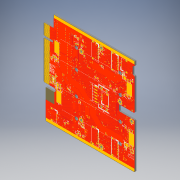
# Autodesk Inventor part: EPS_PCB
Saved by Autodesk Inventor 2018 (Build 220112000, 112)
## iProperties
Created: 2018-01-15
Part Number: EPS_PCB
Material: Epoxy Resin
Document SubType Name: Modeling
Designer: Bradley
Density: 1.14 g/cm^3
Appearance: Smooth - Medium Gray
Mass: 15.4834 g
Surface Area: 175.95 cm^2
Volume: 13.582 cm^3
Author: Bradley
Revision Number: 3.1
Autodesk Inventor part; units mm, degrees
ref_plane "YZ Plane" through (0, 0, 0) normal (1, 0, 0) x (0, 1, 0)
ref_plane "XZ Plane" through (0, 0, 0) normal (0, 1, 0) x (-1, 0, 0)
ref_plane "XY Plane" through (0, 0, 0) normal (0, 0, 1) x (1, 0, 0)
sketch "Sketch1" plane through (0, 0, 0) normal (0, 0, 1) x (1, 0, 0)
  line L0 (0, 36.15) -> (10, 36.15)
  line L1 (10, 36.15) -> (10, 47.9)
  line L2 (10, 47.9) -> (90.4, 47.9)
  line L3 (90.4, 47.9) -> (90.4, -47.9)
  line L4 (90.4, -47.9) -> (2, -47.9)
  line L5 (10, -15.15) -> (0, -15.15)
  line L6 (-5.5, 48) -> (90.5, 48) construction
  line L7 (90.5, 48) -> (90.5, -48) construction
  line L8 (90.5, -48) -> (-5.5, -48) construction
  line L9 (-5.5, -48) -> (-5.5, 48) construction
  line L10 (-5.4, 47.9) -> (-3.4, 47.9) construction
  line L11 (-3.4, 47.9) -> (-3.4, -47.9) construction
  line L12 (-3.4, -47.9) -> (-5.4, -47.9) construction
  line L13 (-5.4, -47.9) -> (-5.4, 47.9) construction
  line L14 (-3.4, 38.5) -> (7.85, 38.5) construction
  line L15 (7.85, 38.5) -> (7.85, -17.5) construction
  line L16 (7.85, -17.5) -> (-3.4, -17.5) construction
  line L17 (-3.4, -17.5) -> (-3.4, 38.5) construction
  line L18 (2, -47.9) -> (2, -18.65)
  line L19 (2, -18.65) -> (10, -18.65)
  arc A0 (10, -18.65) -> (10, -15.15) centre (10, -16.9) ccw
  line L20 (0, 24) -> (90.5, 24) construction
  circle A1 centre (-2.5, 47.1) radius 0.9 construction
  circle A2 centre (-0.7, 47.1) radius 0.9 construction
  circle A3 centre (1.1, 47.1) radius 0.9 construction
  circle A4 centre (2.9, 47.1) radius 0.9 construction
  circle A5 centre (4.7, 47.1) radius 0.9 construction
  circle A6 centre (6.5, 47.1) radius 0.9 construction
  circle A7 centre (8.3, 47.1) radius 0.9 construction
  circle A8 centre (-2.5, 45.3) radius 0.9 construction
  circle A9 centre (-0.7, 45.3) radius 0.9 construction
  circle A10 centre (1.1, 45.3) radius 0.9 construction
  circle A11 centre (2.9, 45.3) radius 0.9 construction
  circle A12 centre (4.7, 45.3) radius 0.9 construction
  circle A13 centre (6.5, 45.3) radius 0.9 construction
  circle A14 centre (8.3, 45.3) radius 0.9 construction
  circle A15 centre (-2.5, 43.5) radius 0.9 construction
  circle A16 centre (-0.7, 43.5) radius 0.9 construction
  circle A17 centre (1.1, 43.5) radius 0.9 construction
  circle A18 centre (2.9, 43.5) radius 0.9 construction
  circle A19 centre (4.7, 43.5) radius 0.9 construction
  circle A20 centre (6.5, 43.5) radius 0.9 construction
  circle A21 centre (8.3, 43.5) radius 0.9 construction
  circle A22 centre (-2.5, 41.7) radius 0.9 construction
  circle A23 centre (-0.7, 41.7) radius 0.9 construction
  circle A24 centre (1.1, 41.7) radius 0.9 construction
  circle A25 centre (2.9, 41.7) radius 0.9 construction
  circle A26 centre (4.7, 41.7) radius 0.9 construction
  circle A27 centre (6.5, 41.7) radius 0.9 construction
  circle A28 centre (8.3, 41.7) radius 0.9 construction
  circle A29 centre (-2.5, 39.9) radius 0.9 construction
  circle A30 centre (-0.7, 39.9) radius 0.9 construction
  circle A31 centre (1.1, 39.9) radius 0.9 construction
  circle A32 centre (2.9, 39.9) radius 0.9 construction
  circle A33 centre (4.7, 39.9) radius 0.9 construction
  circle A34 centre (6.5, 39.9) radius 0.9 construction
  circle A35 centre (8.3, 39.9) radius 0.9 construction
  line L21 (0, 36.15) -> (0, 24.95)
  line L22 (0, 24.95) -> (8.4, 24.95)
  arc A36 (8.4, 23.05) -> (8.4, 24.95) centre (8.4, 24) ccw
  line L23 (8.4, 23.05) -> (0, 23.05)
  line L24 (0, 23.05) -> (0, -15.15)
  point P0 (0, 0)
  point P1 (-5.5, 0)
  point P2 (90.4, 0)
  point P3 (90.5, 0)
  dimension "d0" = 51.3
  dimension "d1" = 95.8
  dimension "d3" = 10
  dimension "d20" = 96
  dimension "d21" = 96
  dimension "d22" = 0.1
  dimension "d23" = 0.1
  dimension "d24" = 2
  dimension "d25" = 0.1
  dimension "d28" = 11.25
  dimension "d29" = 56
  dimension "d31" = 9.5
  dimension "d32" = 30.5
  dimension "d34" = 3.5
  dimension "d35" = 12.15
  dimension "d36" = 39.15
  dimension "d37" = 14.5
  dimension "d38" = 1.15
  dimension "d39" = 1.8
  dimension "d42" = 1.8
  dimension "d45" = 1.8
  dimension "d48" = 2
  dimension "d49" = 3.4
  dimension "d50" = 1.9
  dimension "d51" = 8.4
  dimension "d52" = 24
  constraints: 50 end point, 37 centre point, 11 perpendicular, 7 parallel, 6 point on line, 6 tangent, 5 horizontal, 4 point on circle, 3 midpoint, 3 vertical, 2 collinear, 2 horizontal alignment, 68 other
  measures "d0" distance of L5.end L0.start
  measures "d1" distance of L2.end L3.end
  measures "d3" distance of L0.start L0.end
  measures "d20" distance of L6.start L6.end
  measures "d21" distance of L8.end L6.start
  measures "d22" distance between parallel lines of L2 L6
  measures "d23" distance between parallel lines of L7 L3
  measures "d24" distance between parallel lines of L13 L11
  measures "d25" distance between parallel lines of L13 L9
  measures "d28" distance of L15.end L16.end
  measures "d29" distance of L14.end L15.end
  measures "d31" distance between parallel lines of L14 L6
  measures "d32" distance between parallel lines of L8 L16
  measures "d34" distance between parallel lines of L5 L19
  measures "d35" distance between parallel lines of L20 L0
  measures "d36" distance between parallel lines of L5 L20
  measures "d37" distance between parallel lines of L20 L14
  measures "d38" distance between parallel lines of L19 L16
  measures "d39" diameter of A1
  measures "d42" distance of A1.centre A2.centre
  measures "d45" distance of A1.centre A8.centre
  measures "d48" distance between parallel lines of L18 L24
  measures "d49" distance between parallel lines of L24 L11
  measures "d50" distance between parallel lines of L23 L22
  measures "d51" distance of L21.end L22.end
  measures "d52" distance from line of point (0, 0) L20
extrude "Extrusion1" add sketch "Sketch1" along normal mid plane 1.6
chamfer "Chamfer1" distance 0.5 angle 45 4 edges at (0, 36.15, 0) (0, 24.95, 0) (0, 23.05, 0) (0, -15.15, 0)
fillet "Fillet1" radius 0.5 6 edges at (10, 36.15, 0) (10, 47.9, 0) (90.4, 47.9, 0) (90.4, -47.9, 0) (2, -47.9, 0) (2, -18.65, 0)
sketch "Sketch6" plane through (0, 0, 0.8) normal (0, 0, 1) x (1, 0, 0)
  arc A0 (2.5, -18.65) -> (2, -19.15) centre (2.5, -19.15) ccw projected
  line L0 (2, -19.15) -> (2, -47.4) projected
  arc A1 (2, -47.4) -> (2.5, -47.9) centre (2.5, -47.4) ccw projected
  line L1 (2.5, -47.9) -> (89.9, -47.9) projected
  arc A2 (89.9, -47.9) -> (90.4, -47.4) centre (89.9, -47.4) ccw projected
  line L2 (90.4, -47.4) -> (90.4, 47.4) projected
  arc A3 (90.4, 47.4) -> (89.9, 47.9) centre (89.9, 47.4) ccw projected
  line L3 (89.9, 47.9) -> (10.5, 47.9) projected
  arc A4 (10.5, 47.9) -> (10, 47.4) centre (10.5, 47.4) ccw projected
  line L4 (10, 47.4) -> (10, 36.65) projected
  arc A5 (9.5, 36.15) -> (10, 36.65) centre (9.5, 36.65) ccw projected
  line L5 (9.5, 36.15) -> (0.5, 36.15) projected
  line L6 (0, 35.65) -> (0.5, 36.15) projected
  line L7 (0, 35.65) -> (0, 25.45) projected
  line L8 (0.5, 24.95) -> (0, 25.45) projected
  line L9 (0.5, 24.95) -> (8.4, 24.95) projected
  arc A6 (8.4, 23.05) -> (8.4, 24.95) centre (8.4, 24) ccw projected
  line L10 (8.4, 23.05) -> (0.5, 23.05) projected
  line L11 (0, 22.55) -> (0.5, 23.05) projected
  line L12 (0, 22.55) -> (0, -14.65) projected
  line L13 (0.5, -15.15) -> (0, -14.65) projected
  line L14 (0.5, -15.15) -> (10, -15.15) projected
  arc A7 (10, -18.65) -> (10, -15.15) centre (10, -16.9) ccw projected
  line L15 (10, -18.65) -> (2.5, -18.65) projected
  line L16 (90.4, 47.4) -> (90.4, -47.4) projected
  arc A8 (89.4, 3) -> (90.4, 4) centre (89.4, 4) ccw
  line L17 (89.4, 3) -> (75.9, 3)
  arc A9 (75.9, 3) -> (74.9, 2) centre (75.9, 2) ccw
  line L18 (74.9, 2) -> (74.9, -2)
  arc A10 (74.9, -2) -> (75.9, -3) centre (75.9, -2) ccw
  line L19 (75.9, -3) -> (89.4, -3)
  arc A11 (90.4, -4) -> (89.4, -3) centre (89.4, -4) ccw
  arc A12 (90.4, 34) -> (89.4, 35) centre (89.4, 34) ccw
  arc A13 (88.4, 36) -> (89.4, 35) centre (89.4, 36) ccw
  line L20 (88.4, 36) -> (88.4, 42)
  arc A14 (89.4, 43) -> (88.4, 42) centre (89.4, 42) ccw
  arc A15 (89.4, 43) -> (90.4, 44) centre (89.4, 44) ccw
  point P0 (0, 0)
  point P1 (74.9, 0)
  dimension "d69" = 6
  dimension "d70" = 1
  dimension "d71" = 15.5
  dimension "d81" = 2
  dimension "d82" = 35
  dimension "d83" = 8
  constraints: 16 point on circle, 14 tangent, 8 centre point, 8 end point, 6 equal radius, 4 point on line, 2 perpendicular, 1 horizontal, 1 horizontal alignment, 1 midpoint, 1 vertical, 1 vertical alignment
  measures "d69" distance between parallel lines of L19 L17
  measures "d70" radius of A8
  measures "d71" distance between parallel lines of L2 L18
  measures "d81" distance between parallel lines of L16 L20
  measures "d82" vertical distance of point (0, 0) A12.end
  measures "d83" distance of A12.end A14.start
extrude "Extrusion5" cut sketch "Sketch6" against normal through all contours A11 L19 A10 L18 A9 L17 A8 L2 | A12 A13 L20 A14 A15 L2
sketch "Sketch7" plane through (0, 0, 0.8) normal (0, 0, 1) x (1, 0, 0)
  point P0 (0, 0)
  point P1 (76, -30.5)
  point P2 (32.5, 30.5)
  point P3 (76, 30.5)
  point P4 (76, 11.5)
  point P5 (32.5, 11.5)
  point P6 (76, -11.5)
  point P7 (32.5, -11.5)
  point P8 (32.5, -30.5)
  constraints: 8 other
hole "Hole2" at (76, -30.5, 0.8) at (32.5, 30.5, 0.8) at (76, 30.5, 0.8) at (76, 11.5, 0.8) at (32.5, 11.5, 0.8) at (76, -11.5, 0.8) at (32.5, -11.5, 0.8) at (32.5, -30.5, 0.8) direction (0, 0, -1) diameter 3 end through all
sketch "Sketch8" plane through (0, 0, 0.8) normal (0, 0, 1) x (1, 0, 0)
  point P0 (0, 0)
  point P1 (37.4, -29.6)
  point P2 (57.3, -42.5)
  point P3 (87.4, -5.5)
  point P4 (75.9, 5.5)
  point P5 (37.4, 29.6)
  point P6 (57.3, 42.5)
  constraints: 6 other
hole "Hole3" at (37.4, -29.6, 0.8) at (57.3, -42.5, 0.8) at (87.4, -5.5, 0.8) at (75.9, 5.5, 0.8) at (37.4, 29.6, 0.8) at (57.3, 42.5, 0.8) direction (0, 0, -1) diameter 2.2 end through all
sketch "Sketch9" plane through (0, 0, 0.8) normal (0, 0, 1) x (1, 0, 0)
  point P0 (0, 0)
  point P1 (62.54, 8)
  point P2 (57.46, 8)
  point P3 (62.54, -8)
  point P4 (57.46, -8)
  constraints: 4 other
hole "Hole4" at (62.54, 8, 0.8) at (57.46, 8, 0.8) at (62.54, -8, 0.8) at (57.46, -8, 0.8) direction (0, 0, -1) diameter 1.2 end through all
sketch "Sketch10" plane through (0, 0, 0.8) normal (0, 0, 1) x (1, 0, 0)
  point P0 (0, 0)
  point P1 (7.9, 9.6)
  point P2 (12.3, -3.9)
  constraints: 2 other
hole "Hole5" at (7.9, 9.6, 0.8) at (12.3, -3.9, 0.8) direction (0, 0, -1) diameter 1 end through all
sketch "Sketch11" plane through (0, 0, 0.8) normal (0, 0, 1) x (1, 0, 0)
  point P0 (0, 0)
  point P1 (87.975, 4.15)
  point P2 (80.725, 4.15)
  point P3 (34.1, 39.2)
  point P4 (36.1, -33.4)
  constraints: 4 other
hole "Hole6" at (87.975, 4.15, 0.8) at (80.725, 4.15, 0.8) at (34.1, 39.2, 0.8) at (36.1, -33.4, 0.8) direction (0, 0, -1) diameter 0.7 end through all
sketch "Sketch12" plane through (0, 0, 0.8) normal (0, 0, 1) x (1, 0, 0)
  point P0 (0, 0)
  point P1 (58.431, -41.369)
  point P2 (57.3, -40.9)
  point P3 (56.169, -41.369)
  point P4 (55.7, -42.5)
  point P5 (56.169, -43.631)
  point P6 (57.3, -44.1)
  point P7 (58.431, -43.631)
  point P8 (77.5, 5.5)
  point P9 (77.031, 6.631)
  point P10 (75.9, 7.1)
  point P11 (74.769, 6.631)
  point P12 (74.3, 5.5)
  point P13 (74.769, 4.369)
  point P14 (75.9, 3.9)
  point P15 (77.031, 4.369)
  point P16 (87.4, -3.9)
  point P17 (86.269, -4.369)
  point P18 (85.8, -5.5)
  point P19 (86.269, -6.631)
  point P20 (87.4, -7.1)
  point P21 (88.531, -6.631)
  point P22 (89, -5.5)
  point P23 (39, 29.6)
  point P24 (38.531, 30.731)
  point P25 (37.4, 31.2)
  point P26 (36.269, 30.731)
  point P27 (35.8, 29.6)
  point P28 (36.269, 28.469)
  point P29 (37.4, 28)
  point P30 (39, -29.6)
  point P31 (88.531, -4.369)
  point P32 (58.9, 42.5)
  point P33 (58.431, 43.631)
  point P34 (38.531, -28.469)
  point P35 (56.169, 43.631)
  point P36 (55.7, 42.5)
  point P37 (56.169, 41.369)
  point P38 (57.3, 40.9)
  point P39 (38.531, 28.469)
  point P40 (37.4, -28)
  point P41 (57.3, 44.1)
  point P42 (36.269, -28.469)
  point P43 (35.8, -29.6)
  point P44 (36.269, -30.731)
  point P45 (37.4, -31.2)
  point P46 (38.531, -30.731)
  point P47 (58.9, -42.5)
  point P48 (58.431, 41.369)
  constraints: 48 other
hole "Hole7" at (58.431, -41.369, 0.8) at (57.3, -40.9, 0.8) at (56.169, -41.369, 0.8) at (55.7, -42.5, 0.8) at (56.169, -43.631, 0.8) at (57.3, -44.1, 0.8) at (58.431, -43.631, 0.8) at (77.5, 5.5, 0.8) at (77.031, 6.631, 0.8) at (75.9, 7.1, 0.8) at (74.769, 6.631, 0.8) at (74.3, 5.5, 0.8) at (74.769, 4.369, 0.8) at (75.9, 3.9, 0.8) at (77.031, 4.369, 0.8) at (87.4, -3.9, 0.8) at (86.269, -4.369, 0.8) at (85.8, -5.5, 0.8) at (86.269, -6.631, 0.8) at (87.4, -7.1, 0.8) at (88.531, -6.631, 0.8) at (89, -5.5, 0.8) at (39, 29.6, 0.8) at (38.531, 30.731, 0.8) at (37.4, 31.2, 0.8) at (36.269, 30.731, 0.8) at (35.8, 29.6, 0.8) at (36.269, 28.469, 0.8) at (37.4, 28, 0.8) at (39, -29.6, 0.8) at (88.531, -4.369, 0.8) at (58.9, 42.5, 0.8) at (58.431, 43.631, 0.8) at (38.531, -28.469, 0.8) at (56.169, 43.631, 0.8) at (55.7, 42.5, 0.8) at (56.169, 41.369, 0.8) at (57.3, 40.9, 0.8) at (38.531, 28.469, 0.8) at (37.4, -28, 0.8) at (57.3, 44.1, 0.8) at (36.269, -28.469, 0.8) at (35.8, -29.6, 0.8) at (36.269, -30.731, 0.8) at (37.4, -31.2, 0.8) at (38.531, -30.731, 0.8) at (58.9, -42.5, 0.8) at (58.431, 41.369, 0.8) direction (0, 0, -1) diameter 0.35 end through all
sketch "Sketch13" plane through (0, 0, 0.8) normal (0, 0, 1) x (1, 0, 0)
  point P0 (0, 0)
  point P1 (13.9, 37.7)
  point P2 (13.9, 41.7)
  point P3 (13.9, 33.7)
  point P4 (13.9, 29.7)
  point P5 (16, 25.7)
  point P6 (16, 21.7)
  point P7 (16, 17.7)
  point P8 (15.9, 13.7)
  point P9 (16, 9.7)
  point P10 (15.9, 5.7)
  point P11 (23.7, 3.7)
  point P12 (23.7, 7.7)
  point P13 (23.915, 11.745)
  point P14 (23.7, 15.7)
  point P15 (23.765, 19.74)
  point P16 (23.7, 23.7)
  point P17 (23.7, 27.7)
  point P18 (21.69, 31.695)
  point P19 (21.7, 35.7)
  point P20 (21.7, 39.7)
  point P21 (10.29, 10.02)
  point P22 (12.8, -10.8)
  point P23 (37.7, 36.5)
  point P24 (52.5, 35.9)
  point P25 (51.3, 31.8)
  point P26 (51.4, 43.8)
  point P27 (51.4, 43)
  point P28 (51.4, 42.2)
  point P29 (52.2, 42.2)
  point P30 (35.2, 40.4)
  point P31 (35.2, 39.6)
  point P32 (35.2, 38.8)
  point P33 (36.9, 40.4)
  point P34 (36.9, 39.6)
  point P35 (36.9, 38.8)
  point P36 (39.7, 31.6)
  point P37 (39.7, 30.8)
  point P38 (41.8, 35.2)
  point P39 (42.1, 35.8)
  point P40 (41.8, 36.4)
  point P41 (40.8, 36.5)
  point P42 (39.8, 36.4)
  point P43 (39.5, 35.8)
  point P44 (39.8, 35.2)
  point P45 (43.2, 19.5)
  point P46 (43.2, 20.7)
  point P47 (44.8, 19.5)
  point P48 (44, 19.5)
  point P49 (40.5, 31.6)
  point P50 (40.5, 30)
  point P51 (57.2, 36)
  point P52 (57.2, 38.9)
  point P53 (64.8, 40.7)
  point P54 (61.95, 43.2)
  point P55 (59.3, 30.1)
  point P56 (68.2, 36.7)
  point P57 (71, 36.7)
  point P58 (73.5, 33)
  point P59 (63.6, 30.8)
  point P60 (64.2, 32.9)
  point P61 (66.6, 31.9)
  point P62 (69.7, 29.7)
  point P63 (10.6, 42)
  point P64 (22, 18.695)
  point P65 (22, 9.7)
  point P66 (29.47, 15.2)
  point P67 (40, 22.6)
  point P68 (35.3, 27.2)
  point P69 (39.4, 27.1)
  point P70 (46.6, -43.1)
  point P71 (46.6, -44.4)
  point P72 (47.4, -44.4)
  point P73 (47.4, -43.7)
  point P74 (47.4, -43)
  point P75 (46.6, -43.7)
  point P76 (42.2, -37.8)
  point P77 (41.6, -37.8)
  point P78 (41, -37.8)
  point P79 (40.9, -38.8)
  point P80 (41, -39.8)
  point P81 (41.6, -40.1)
  point P82 (42.2, -39.8)
  point P83 (41.6, -35.4)
  point P84 (42.4, -35.4)
  point P85 (43.2, -35.4)
  point P86 (42.4, -37.1)
  point P87 (41.7, -37.1)
  point P88 (50.2, -28.8)
  point P89 (51, -28.8)
  point P90 (51.8, -28.8)
  point P91 (52.6, -28.8)
  point P92 (52.6, -28)
  point P93 (52.6, -27.2)
  point P94 (53.1, -31.5)
  point P95 (57.6, -40)
  point P96 (64.8, -42.9)
  point P97 (64.7, -39.8)
  point P98 (73.8, -42.9)
  point P99 (73.5, -40.62)
  point P100 (68.2, -38.9)
  point P101 (64.7, -34.7)
  point P102 (70.1, -34.7)
  point P103 (60, -34.6)
  point P104 (12, -41.3)
  point P105 (6.7, -40.65)
  point P106 (79.8, -31.7)
  point P107 (84.6, -33)
  point P108 (59.1, -32.9)
  point P109 (82.75, -5.8)
  point P110 (89.4, -37.7)
  point P111 (54, 33)
  point P112 (77.9, 41.2)
  point P113 (77.7, 35)
  point P114 (43.2, 20.1)
  point P115 (45.6, 20.1)
  point P116 (83.2, 10.9)
  point P117 (78.415, 10.635)
  point P118 (82, 13.8)
  point P119 (58, 1.5)
  point P120 (35.7, -24.95)
  point P121 (38.2, -15.4)
  point P122 (45.6, 19.5)
  point P123 (52.2, 43)
  point P124 (41, -36.2)
  point P125 (41, -37)
  point P126 (6.1, 11.1)
  point P127 (6.1, 10.3)
  point P128 (6.1, 9.5)
  point P129 (6.1, 8.7)
  point P130 (6.1, 7.9)
  point P131 (6.1, 7.1)
  point P132 (6.1, 6.3)
  point P133 (6.1, 5.5)
  point P134 (78.29, -34.2)
  point P135 (87.1, 36.4)
  point P136 (77.34, 13.12)
  point P137 (71.66, -8.115)
  point P138 (85.155, -30.25)
  point P139 (72.8, -18.24)
  point P140 (72.76, -19.96)
  point P141 (78.29, -35)
  point P142 (87.095, 35.64)
  point P143 (77.335, 13.88)
  point P144 (71.4, -7.4)
  point P145 (85.155, -31.015)
  point P146 (72.04, -18.24)
  point P147 (72, -19.96)
  point P148 (81.78, -23.295)
  point P149 (66, -2.185)
  point P150 (69.9, -2.2)
  point P151 (56.6, 33.9)
  point P152 (70, 28.3)
  point P153 (68.4, 33.9)
  point P154 (62, 39.1)
  point P155 (60.9, 32.5)
  point P156 (71.39, -36.73)
  point P157 (62.5, -35.8)
  point P158 (62.8, -39.2)
  point P159 (67.1, -32.9)
  point P160 (81.5, 15.2)
  point P161 (81.8, 16.99)
  point P162 (81.2, 16.99)
  point P163 (80.6, 16.99)
  point P164 (81.8, 17.59)
  point P165 (81.2, 17.59)
  point P166 (82.1, 15.2)
  point P167 (82.1, 14.6)
  point P168 (81.5, 14.6)
  point P169 (68.2, 2)
  point P170 (56.4, 36.81)
  point P171 (62, 33.1)
  point P172 (69, 28.1)
  point P173 (74.5, 37.3)
  point P174 (71.18, 27.71)
  point P175 (72.5, 34.9)
  point P176 (72, 27.6)
  point P177 (58, -36.75)
  point P178 (38.7, -35.5)
  point P179 (59.1, -39.8)
  point P180 (38.7, -41.5)
  point P181 (75, -37.9)
  point P182 (37.8, -35.6)
  point P183 (75.5, -41.6)
  point P184 (70.2, -37.9)
  point P185 (37.86, -38.715)
  point P186 (68.5, 37.65)
  point P187 (66.3, -43.2)
  point P188 (66.3, -36.73)
  point P189 (84.3, -15)
  point P190 (82.7, -15.8)
  point P191 (83.5, -15.8)
  point P192 (83.5, -15)
  point P193 (84.3, -14.2)
  point P194 (83.5, -14.2)
  point P195 (82.7, -15)
  point P196 (82.7, -14.2)
  point P197 (65.6, 33.5)
  point P198 (84.5, 13.8)
  point P199 (70.7, -4.8)
  constraints: 687 other
hole "Hole8" at (13.9, 37.7, 0.8) at (13.9, 41.7, 0.8) at (13.9, 33.7, 0.8) at (13.9, 29.7, 0.8) at (16, 25.7, 0.8) at (16, 21.7, 0.8) at (16, 17.7, 0.8) at (15.9, 13.7, 0.8) at (16, 9.7, 0.8) at (15.9, 5.7, 0.8) at (23.7, 3.7, 0.8) at (23.7, 7.7, 0.8) at (23.915, 11.745, 0.8) at (23.7, 15.7, 0.8) at (23.765, 19.74, 0.8) at (23.7, 23.7, 0.8) at (23.7, 27.7, 0.8) at (21.69, 31.695, 0.8) at (21.7, 35.7, 0.8) at (21.7, 39.7, 0.8) at (10.29, 10.02, 0.8) at (12.8, -10.8, 0.8) at (37.7, 36.5, 0.8) at (52.5, 35.9, 0.8) at (51.3, 31.8, 0.8) at (51.4, 43.8, 0.8) at (51.4, 43, 0.8) at (51.4, 42.2, 0.8) at (52.2, 42.2, 0.8) at (35.2, 40.4, 0.8) at (35.2, 39.6, 0.8) at (35.2, 38.8, 0.8) at (36.9, 40.4, 0.8) at (36.9, 39.6, 0.8) at (36.9, 38.8, 0.8) at (39.7, 31.6, 0.8) at (39.7, 30.8, 0.8) at (41.8, 35.2, 0.8) at (42.1, 35.8, 0.8) at (41.8, 36.4, 0.8) at (40.8, 36.5, 0.8) at (39.8, 36.4, 0.8) at (39.5, 35.8, 0.8) at (39.8, 35.2, 0.8) at (43.2, 19.5, 0.8) at (43.2, 20.7, 0.8) at (44.8, 19.5, 0.8) at (44, 19.5, 0.8) at (40.5, 31.6, 0.8) at (40.5, 30, 0.8) direction (0, 0, -1) diameter 0.3 end through all and at (57.2, 36, 0.8) (57.2, 38.9, 0.8) (64.8, 40.7, 0.8) (61.95, 43.2, 0.8) (59.3, 30.1, 0.8) (68.2, 36.7, 0.8) (71, 36.7, 0.8) (73.5, 33, 0.8) (63.6, 30.8, 0.8) (64.2, 32.9, 0.8) (66.6, 31.9, 0.8) (69.7, 29.7, 0.8) (10.6, 42, 0.8) (22, 18.695, 0.8) (22, 9.7, 0.8) (29.47, 15.2, 0.8) (40, 22.6, 0.8) (35.3, 27.2, 0.8) (39.4, 27.1, 0.8) (46.6, -43.1, 0.8) (46.6, -44.4, 0.8) (47.4, -44.4, 0.8) (47.4, -43.7, 0.8) (47.4, -43, 0.8) (46.6, -43.7, 0.8) (42.2, -37.8, 0.8) (41.6, -37.8, 0.8) (41, -37.8, 0.8) (40.9, -38.8, 0.8) (41, -39.8, 0.8) (41.6, -40.1, 0.8) (42.2, -39.8, 0.8) (41.6, -35.4, 0.8) (42.4, -35.4, 0.8) (43.2, -35.4, 0.8) (42.4, -37.1, 0.8) (41.7, -37.1, 0.8) (50.2, -28.8, 0.8) (51, -28.8, 0.8) (51.8, -28.8, 0.8) (52.6, -28.8, 0.8) (52.6, -28, 0.8) (52.6, -27.2, 0.8) (53.1, -31.5, 0.8) (57.6, -40, 0.8) (64.8, -42.9, 0.8) (64.7, -39.8, 0.8) (73.8, -42.9, 0.8) (73.5, -40.62, 0.8) (68.2, -38.9, 0.8) (64.7, -34.7, 0.8) (70.1, -34.7, 0.8) (60, -34.6, 0.8) (12, -41.3, 0.8) (6.7, -40.65, 0.8) (79.8, -31.7, 0.8) (84.6, -33, 0.8) (59.1, -32.9, 0.8) (82.75, -5.8, 0.8) (89.4, -37.7, 0.8) (54, 33, 0.8) (77.9, 41.2, 0.8) (77.7, 35, 0.8) (43.2, 20.1, 0.8) (45.6, 20.1, 0.8) (83.2, 10.9, 0.8) (78.415, 10.635, 0.8) (82, 13.8, 0.8) (58, 1.5, 0.8) (35.7, -24.95, 0.8) (38.2, -15.4, 0.8) (45.6, 19.5, 0.8) (52.2, 43, 0.8) (41, -36.2, 0.8) (41, -37, 0.8) (6.1, 11.1, 0.8) (6.1, 10.3, 0.8) (6.1, 9.5, 0.8) (6.1, 8.7, 0.8) (6.1, 7.9, 0.8) (6.1, 7.1, 0.8) (6.1, 6.3, 0.8) (6.1, 5.5, 0.8) (78.29, -34.2, 0.8) (87.1, 36.4, 0.8) (77.34, 13.12, 0.8) (71.66, -8.115, 0.8) (85.155, -30.25, 0.8) (72.8, -18.24, 0.8) (72.76, -19.96, 0.8) (78.29, -35, 0.8) (87.095, 35.64, 0.8) (77.335, 13.88, 0.8) (71.4, -7.4, 0.8) (85.155, -31.015, 0.8) (72.04, -18.24, 0.8) (72, -19.96, 0.8) (81.78, -23.295, 0.8) (66, -2.185, 0.8) (69.9, -2.2, 0.8) (56.6, 33.9, 0.8) (70, 28.3, 0.8) (68.4, 33.9, 0.8) (62, 39.1, 0.8) (60.9, 32.5, 0.8) (71.39, -36.73, 0.8) (62.5, -35.8, 0.8) (62.8, -39.2, 0.8) (67.1, -32.9, 0.8) (81.5, 15.2, 0.8) (81.8, 16.99, 0.8) (81.2, 16.99, 0.8) (80.6, 16.99, 0.8) (81.8, 17.59, 0.8) (81.2, 17.59, 0.8) (82.1, 15.2, 0.8) (82.1, 14.6, 0.8) (81.5, 14.6, 0.8) (68.2, 2, 0.8) (56.4, 36.81, 0.8) (62, 33.1, 0.8) (69, 28.1, 0.8) (74.5, 37.3, 0.8) (71.18, 27.71, 0.8) (72.5, 34.9, 0.8) (72, 27.6, 0.8) (58, -36.75, 0.8) (38.7, -35.5, 0.8) (59.1, -39.8, 0.8) (38.7, -41.5, 0.8) (75, -37.9, 0.8) (37.8, -35.6, 0.8) (75.5, -41.6, 0.8) (70.2, -37.9, 0.8) (37.86, -38.715, 0.8) (68.5, 37.65, 0.8) (66.3, -43.2, 0.8) (66.3, -36.73, 0.8) (84.3, -15, 0.8) (82.7, -15.8, 0.8) (83.5, -15.8, 0.8) (83.5, -15, 0.8) (84.3, -14.2, 0.8) (83.5, -14.2, 0.8) (82.7, -15, 0.8) (82.7, -14.2, 0.8) (65.6, 33.5, 0.8) (84.5, 13.8, 0.8) (70.7, -4.8, 0.8) (83.355, -3.96, 0.8) (77, 37.5, 0.8) (5.3, -38.3, 0.8) (18.7, -43.7, 0.8) (81.7, -33.4, 0.8) (87.2, -34.6, 0.8) (67.3, 19.215, 0.8) (65.34, 16.795, 0.8) (58.84, -22.08, 0.8) (71.54, -11.46, 0.8) (53.71, -6.57, 0.8) (68, 18.915, 0.8) (65.88, 16.255, 0.8) (58.08, -22.08, 0.8) (71.76, -12.19, 0.8) (54.345, -6.99, 0.8) (69.5, 19.215, 0.8) (66.96, 15.175, 0.8) (72.94, -11.7, 0.8) (59.17, -23.16, 0.8) (53.89, -5.83, 0.8) (68.8, 18.915, 0.8) (66.42, 15.715, 0.8) (59.93, -23.17, 0.8) (72.62, -11.01, 0.8) (54.57, -5.49, 0.8) (8.09, -8.99, 0.8) (6.2, -11.2, 0.8) (22.4, -12.1, 0.8) (22.4, -15, 0.8) (29.8, 34.1, 0.8) (34.9, 32.9, 0.8) (36.025, 15.595, 0.8) (28.5, -39.9, 0.8) (29.2, -42.7, 0.8) (13.9, -44, 0.8) (80.1, -35.8, 0.8) (77.395, -37.24, 0.8) (80.3, -11.5, 0.8) (78.1, -11.1, 0.8) (61.465, -22.4, 0.8) (47.7, 6.3, 0.8) (36.1, 2.8, 0.8) (22.6, -0.4, 0.8) (77.6, 23.5, 0.8) (63.7, 13.27, 0.8) (51.395, 20.445, 0.8) (44.8, 13.3, 0.8) (46.1, -10.8, 0.8) (38.1, -9.9, 0.8) (50.3, 2, 0.8) (61.82, -4.17, 0.8) (44.5, -14.6, 0.8) (24.9, -17.7, 0.8) (28.4, -18.5, 0.8) (64.69, 33.91, 0.8) (55.96, 26.7, 0.8) (39.3, -25.44, 0.8) (20.7, -36.8, 0.8) (16, 14.5, 0.8) (16, 10.5, 0.8) (16, 6.5, 0.8) (23.8, 4.5, 0.8) (23.8, 8.5, 0.8) (23.8, 12.5, 0.8) (23.8, 16.5, 0.8) (27.1, 15.2, 0.8) (52.3, -41.5, 0.8) (53, -41.5, 0.8) (53, -42.3, 0.8) (55, -40.3, 0.8) (55.8, -40.3, 0.8) (55, -41.1, 0.8) (62.8, -29, 0.8) (62.8, -29.8, 0.8) (61.9, -29.8, 0.8) (61.9, -29, 0.8) (61.9, -28.2, 0.8) (61.1, -29, 0.8) (61.1, -28.2, 0.8) (81.5, -26.1, 0.8) (81.2, 25.9, 0.8) (61, 12.46, 0.8) (51.3, -13.2, 0.8) (4.3, -36.6, 0.8) (61.1, -29.8, 0.8) (52.3, -42.3, 0.8) (53.8, -42.3, 0.8) (11.795, 7.67, 0.8) (12.3, 7.1, 0.8) (16, 15.98, 0.8) (15.995, 11.98, 0.8) (16, 7.98, 0.8) (23.8, 6, 0.8) (23.8, 10, 0.8) (23.8, 14, 0.8) (23.9, 18, 0.8) (45.9, 25, 0.8) (46.7, 25, 0.8) (47.5, 25, 0.8) (48.3, 25, 0.8) (48.3, 25.8, 0.8) (48.3, 26.6, 0.8) (82, -4.3, 0.8) (73.9, 28.4, 0.8) (64.22, 18.4, 0.8) (6.8, -39.2, 0.8) (13.7, 4.4, 0.8) (56.315, 27.375, 0.8) (40.7, -42.7, 0.8) (34.9, -39.7, 0.8) (83.9, -22.5, 0.8) (83.9, -17.2, 0.8) (82.4, -25.6, 0.8) (20.9, -41.7, 0.8) (24, -42.8, 0.8) (36.2, -35.4, 0.8) (81.9, 23.3, 0.8) (44.1, 22.1, 0.8) (54.4, 15.9, 0.8) (52.5, 14.6, 0.8) (26.7, -4.3, 0.8) (46.3, 19.8, 0.8) (71.18, 17.96, 0.8) (75.1, 17.3, 0.8) (71.66, 12.95, 0.8) (61, 18.735, 0.8) (65.465, 13.585, 0.8) (71.28, -18.24, 0.8) (36, 4.7, 0.8) (50.4, 11.1, 0.8) (89.8, 14.2, 0.8) (83, -24.1, 0.8) (82.2, -24.1, 0.8) (85.2, 28.9, 0.8) (84.4, 28.9, 0.8) (85.6, -29.1, 0.8) (88.6, 28.4, 0.8) (88.4, 13, 0.8) (81, 31.3, 0.8) (81.5, -31.5, 0.8) (87.2, -28.8, 0.8) (86.4, -28.8, 0.8) (88.3, -31.1, 0.8) (88.2, -12.7, 0.8) (87.4, -12.7, 0.8) (15.4, -11, 0.8) (15.4, -12.6, 0.8) (17, -12.91, 0.8) (15.45, -35.315, 0.8) (89.4, -31.4, 0.8) (87.3, 12.1, 0.8) (85.6, 12.1, 0.8) (69.8, 2.8, 0.8) (79.6, 11.8, 0.8) (5.9, -5.5, 0.8) (39.69, -0.55, 0.8) (78.82, 13.46, 0.8) (41.7, 39.2, 0.8) (14, 44, 0.8) (14.005, 39.975, 0.8) (14, 35.98, 0.8) (14.005, 31.98, 0.8) (16.005, 27.98, 0.8) (16, 23.98, 0.8) (16, 19.98, 0.8) (23.9, 22, 0.8) (23.8, 26, 0.8) (21.8, 34, 0.8) (21.8, 38, 0.8) (21.8, 42, 0.8) (23.58, 30.6, 0.8) (37.5, 42.4, 0.8) (36.7, 42.4, 0.8) (36.7, 43.2, 0.8) (37.5, 43.2, 0.8) (37.5, 41.6, 0.8) (36.7, 41.6, 0.8) (58.69, 28.175, 0.8) (48.935, 19.86, 0.8) (44.92, 10.98, 0.8) (57.11, -21.28, 0.8) (38.9, 2.5, 0.8) (38.9, 4.2, 0.8) (49.9, -10.235, 0.8) (83, -37, 0.8) (89.2, -34.7, 0.8) (14, 42.5, 0.8) (14, 38.5, 0.8) (14, 34.5, 0.8) (14, 30.5, 0.8) (16, 26.5, 0.8) (16, 22.5, 0.8) (16, 18.5, 0.8) (23.815, 20.5, 0.8) (23.8, 24.5, 0.8) (23.8, 28.5, 0.8) (21.765, 32.54, 0.8) (21.8, 36.5, 0.8) (21.8, 40.5, 0.8) (13, 44.4, 0.8) (42.9, -22.6, 0.8) (42.3, -22.9, 0.8) (43.7, -22.6, 0.8) (43.7, -23.4, 0.8) (43.7, -24.2, 0.8) (88, -34.7, 0.8) (18.5, 1.1, 0.8) (19.3, 1.1, 0.8) (20.1, 1.1, 0.8) (20.1, 0.3, 0.8) (19.3, 0.3, 0.8) (18.5, 0.3, 0.8) (18.5, -0.5, 0.8) (19.3, -0.5, 0.8) (42.295, -15.04, 0.8) (44.5, -22.6, 0.8) (44.5, -23.4, 0.8) (44.5, -24.2, 0.8) (45.3, -24.2, 0.8) (45.3, -23.4, 0.8) (45.3, -22.6, 0.8) (42.9, -27.9, 0.8) (39.9, -33.9, 0.8) (30, 39.4, 0.8) (74.765, 16.16, 0.8) (72.8, 16.2, 0.8) (39.2, -44, 0.8) (32.1, -44.4, 0.8) (28.855, -9.895, 0.8) (30.815, -16.8, 0.8) (39.98, -26.8, 0.8) (17.6, -37.7, 0.8) (5.9, 35.5, 0.8) (9.55, -9.34, 0.8) (10.1, -6.5, 0.8) (5.9, 34.5, 0.8) (12.1, 40.835, 0.8) (5.9, 33.5, 0.8) (11.7, 39.45, 0.8) (5.9, 32.5, 0.8) (5.9, 31.5, 0.8) (5.9, 30.5, 0.8) (5.9, 29.5, 0.8) (5.9, 28.5, 0.8) (5.9, 27.5, 0.8) (5.9, 26.5, 0.8) (5.9, 25.6, 0.8) (9.3, 25.5, 0.8) (5.9, 22.4, 0.8) (9.1, 22.5, 0.8) (5.9, 21.5, 0.8) (28.03, 40.835, 0.8) (33.84, 20.76, 0.8) (27.615, 38.87, 0.8) (33.67, 20.015, 0.8) (25.8, 39.1, 0.8) (32.76, 20.76, 0.8) (25.9, 36.7, 0.8) (32, 20.76, 0.8) (25.8, 35.1, 0.8) (31.87, 20.01, 0.8) (25.8, 31.1, 0.8) (32.37, 17.98, 0.8) (27.9, 28.7, 0.8) (32.19, 15.57, 0.8) (28.095, 26.88, 0.8) (32.49, 14.87, 0.8) (27.9, 24.7, 0.8) (32.01, 14.28, 0.8) (27.8, 23.1, 0.8) (33.8, 9.5, 0.8) (27.89, 20.7, 0.8) (30.03, 12.85, 0.8) (26.9, 19.2, 0.8) (33.165, 9.08, 0.8) (29.9, 18, 0.8) (41.53, 21.79, 0.8) (25.9, 32.7, 0.8) (31.87, 19.245, 0.8) (34.67, 7.705, 0.8) (29.71, 3.92, 0.8) (18.44, -2.79, 0.8) (20.29, -10.94, 0.8) (28.315, -9.36, 0.8) (31.88, -25.3, 0.8) (63.455, -20.64, 0.8) (46.1, -6.8, 0.8) (27.9, 16.7, 0.8) (29.71, 11.64, 0.8) (5.9, 20.5, 0.8) (5.9, 19.5, 0.8) (25.9, 15.1, 0.8) (29.68, 10.88, 0.8) (5.9, 18.5, 0.8) (27.89, 12.5, 0.8) (28.96, 10.535, 0.8) (28.2, 10.6, 0.8) (30.67, 8.36, 0.8) (34.8, -43.4, 0.8) (27.9, 8.7, 0.8) (30.93, 7.645, 0.8) (5.9, 16.5, 0.8) (27.8, 7.3, 0.8) (30.67, 6.93, 0.8) (5.9, 15.5, 0.8) (27.9, 4.7, 0.8) (45.85, 4.725, 0.8) (5.9, 14.5, 0.8) (60, 3.5, 0.8) (46.6, 2.4, 0.8) (31.03, 2.045, 0.8) (60.54, 5.13, 0.8) (29.395, -9.36, 0.8) (31.58, -16.8, 0.8) (55.7, -15.63, 0.8) (55.7, -14.5, 0.8) (81.79, 24.055, 0.8) (48.485, 0.89, 0.8) (66.69, 5.48, 0.8) (68.7, 10.4, 0.8) (81.9, 26.3, 0.8) (62.6, 19.84, 0.8) (28.7, 39.8, 0.8) (30.03, 30.83, 0.8) (40.01, 0.9, 0.8) (39.69, 0.21, 0.8) (41.41, 0.69, 0.8) (11.9, -15.4, 0.8) (18.7, -10.605, 0.8) (18.2, -16.5, 0.8) (18.7, -14.1, 0.8) (5.9, -9.5, 0.8) (5.9, -8.5, 0.8) (5.9, -10.5, 0.8) (41.09, 0, 0.8) (27.6, -14.51, 0.8) (24.875, -10.94, 0.8) (5.9, -7.5, 0.8) (33.9, 32.1, 0.8) (35.36, 18.425, 0.8) (15.01, -42.2, 0.8) (50.95, 18.78, 0.8) (19.26, -3.56, 0.8) (31.34, -25.84, 0.8) (51.675, -11.495, 0.8) (58, -20.64, 0.8) (34.66, 32.175, 0.8) (36.14, 18.41, 0.8) (15.21, -43.025, 0.8) (51.44, 19.365, 0.8) (19.525, -4.275, 0.8) (30.62, -26.105, 0.8) (52.215, -10.96, 0.8) (58.69, -20.96, 0.8) (48.5, -1.81, 0.8) (54.885, -4.415, 0.8) (12.3, -7.8, 0.8) (27.195, -9.92, 0.8) (28.285, -14.12, 0.8) (76.87, 18.35, 0.8) (71.62, 10.405, 0.8) (77.1, -18.7, 0.8) (74.02, -18.435, 0.8) (76.33, 18.885, 0.8) (71.62, 9.63, 0.8) (77.1, -17.9, 0.8) (73.48, -17.9, 0.8) (27.66, -34.62, 0.8) (28.44, -33.87, 0.8) (28.44, -32.03, 0.8) (77.41, 18.885, 0.8) (72.38, 10.4, 0.8) (77.1, -19.5, 0.8) (74.56, -18.975, 0.8) (28.12, -33.18, 0.8) (26.94, -34.355, 0.8) (50.5, 7.1, 0.8) (35.36, -13.43, 0.8) (16.1, -35.72, 0.8) (12.3, -9.4, 0.8) (28.9, -13.205, 0.8) (26.715, -10.94, 0.8) (12.3, -8.6, 0.8) (29.44, -12.665, 0.8) (27.475, -10.94, 0.8) (12.3, -10.2, 0.8) (29.44, -13.745, 0.8) (25.955, -10.94, 0.8) (36.65, -41.35, 0.8) (81.9, 22.5, 0.8) (77.95, 18.35, 0.8) (56.99, 5.41, 0.8) (5.9, 17.5, 0.8) (74.66, -17.095, 0.8) (48.4, -3, 0.8) (38.3, 36, 0.8) (40.95, 23.5, 0.8) (27.195, -8.84, 0.8) (57.3, 13.8, 0.8) (22, -40, 0.8) (61.67, 19.095, 0.8) (50.28, 18.42, 0.8) (25.2, -38.3, 0.8) (18.46, -4.74, 0.8) (14.2, -34.58, 0.8) (64.22, 34.51, 0.8) (56.72, 26.73, 0.8) (38.76, -24.905, 0.8) (14.96, -35.9, 0.8) (71.4, -31.6, 0.8) (63.735, -31.04, 0.8) (28.525, 3.19, 0.8) (40.1, -20.565, 0.8) (28.255, -10.955, 0.8) (87.7, -33.2, 0.8) (30.5, -43.4, 0.8) (40.7, -44, 0.8) (34.4, -38, 0.8) (34.5, -35.8, 0.8) (31.7, -33.7, 0.8) (22.1, -43.9, 0.8) (9.7, -43.3, 0.8) (39.66, -26.11, 0.8) (20, -37.1, 0.8) (18.72, -5.455, 0.8) (36.075, -13.17, 0.8) (70.6, -31.6, 0.8) (59.9, -31.6, 0.8) (86, -12.4, 0.8) (89.2, -12.4, 0.8) (78.9, -21.3, 0.8) (83.5, -21.8, 0.8) (81.4, -22.6, 0.8) (83.6, -26, 0.8) (84.8, -29.1, 0.8) (29.2, 18.3, 0.8) (29.2, 39.2, 0.8) (30.03, 31.595, 0.8) (63.68, 35.415, 0.8) (82, 18.7, 0.8) (78.71, 18.4, 0.8) (70.1, 24.7, 0.8) (73, 21.9, 0.8) (55.56, 27.69, 0.8) (57.5, 16, 0.8) (42.73, 22.395, 0.8) (29.6, -4.4, 0.8) (71.9, 18.8, 0.8) (71.79, 13.7, 0.8) (42.638, 24.252, 0.8) (55.9, 13.9, 0.8) (67.69, 14.95, 0.8) (88.44, 15.85, 0.8) (81.1, -12.3, 0.8) (78.18, -10.195, 0.8) (81.1, -6.7, 0.8) (71.46, -20.495, 0.8) (6.475, -9, 0.8) (6.475, -7, 0.8) (20.6, -14.5, 0.8) (20.6, -17.3, 0.8) (17.7, -11.2, 0.8) (31.1, 33.25, 0.8) (36.4, -40.4, 0.8) (29.4, -39.5, 0.8) (80.4, -15.3, 0.8) (80.1, -33.8, 0.8) (83.5, -20.09, 0.8) (46.9, 6.3, 0.8) (36, 1.1, 0.8) (23.9, -1.6, 0.8) (52.3, 16.9, 0.8) (37.1, 16.6, 0.8) (79, 24.8, 0.8) (21.1, -42.5, 0.8) (55.95, 2.9, 0.8) (57, -2.2, 0.8) (48.4, -3.8, 0.8) (47.5, -10.8, 0.8) (39.71, -9.9, 0.8) (54, 5.6, 0.8) (22.375, -7.815, 0.8) (53.9, 1, 0.8) (6.1, 13.5, 0.8) (6.1, 12.7, 0.8) (6.1, 11.9, 0.8) (82.985, -17.14, 0.8)
sketch "Sketch14" plane through (0, 0, 0.8) normal (0, 0, 1) x (1, 0, 0)
  line L0 (0, 22.55) -> (0, -14.65) projected
  line L1 (90.4, 4) -> (90.4, 34) projected
  line L2 (0, 47.8927) -> (90.4, 47.8927) construction
  line L3 (90.4, 47.8927) -> (90.4, -47.8927) construction
  line L4 (90.4, -47.8927) -> (0, -47.8927) construction
  line L5 (0, -47.8927) -> (0, 47.8927) construction
  point P0 (0, 0)
  constraints: 2 collinear, 1 midpoint, 2 other
decal "Decal1"
sketch "Sketch15" plane through (0, 0, -0.8) normal (0, 0, -1) x (-1, 0, 0)
  line L0 (-90.4, 34) -> (-90.4, 4) projected
  line L1 (0, -14.65) -> (0, 22.55) projected
  line L2 (-90.4, 47.8927) -> (0, 47.8927) construction
  line L3 (0, 47.8927) -> (0, -47.8927) construction
  line L4 (0, -47.8927) -> (-90.4, -47.8927) construction
  line L5 (-90.4, -47.8927) -> (-90.4, 47.8927) construction
  point P0 (0, 0)
  constraints: 2 collinear, 1 midpoint, 2 other
decal "Decal2"
equation "\"d23\" = d22"
equation "\"d25\" = d22"
equation "\"d42\" = d39"
equation "\"d45\" = d39"
body "Solid1"
